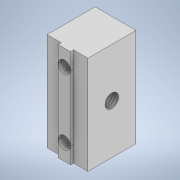
# Autodesk Inventor part: elbow clamp
Saved by Autodesk Inventor 2021 (Build 250183000, 183)
## iProperties
Created: 2022-09-09
Part Number: elbow clamp
Material: Generic
Document SubType Name: Modeling
Designer: szucs
Density: 1 g/cm^3
Appearance: Default
Author: szucs
Autodesk Inventor part; units mm, degrees
ref_plane "YZ Plane" through (0, 0, 0) normal (1, 0, 0) x (0, 1, 0)
ref_plane "XZ Plane" through (0, 0, 0) normal (0, 1, 0) x (-1, 0, 0)
ref_plane "XY Plane" through (0, 0, 0) normal (0, 0, 1) x (1, 0, 0)
sketch "Sketch1" plane through (0, 0, 0) normal (0, 0, 1) x (1, 0, 0)
  line L0 (0, 33.6) -> (0, -33.6) projected
  line L1 (-14, 0) -> (14, 0) projected
  line L2 (-10, 24) -> (10, 24)
  line L3 (10, 24) -> (10, -24)
  line L4 (10, -24) -> (-10, -24)
  line L5 (-10, -24) -> (-10, 24)
  point P0 (0, 0)
  dimension "d0" = 20
  dimension "d1" = 48
  constraints: 8 end point, 2 parallel, 1 horizontal, 1 perpendicular, 2 other
  measures "d0" distance of L3.end L4.end
  measures "d1" distance of L2.end L3.end
extrude "Extrusion1" add sketch "Sketch1" along normal blind 25
sketch "Sketch2" plane through (0, 0, 25) normal (0, 0, 1) x (1, 0, 0)
  line L0 (-10, -24) -> (10, -24) projected
  line L1 (10, -24) -> (10, 24) projected
  line L2 (10, 24) -> (-10, 24) projected
  line L3 (-10, 24) -> (-10, -24) projected
  line L4 (0, 47.04) -> (0, -47.04) projected
  line L5 (3, 33.6) -> (3, -33.6)
  line L6 (-3, 33.6) -> (-3, -33.6)
  point P0 (0, 0)
  point P1 (3, 24)
  point P2 (3, -24)
  point P3 (-3, -24)
  point P4 (-3, 24)
  dimension "d4" = 3
  dimension "d5" = 3
  constraints: 4 end point, 2 parallel
  measures "d4" distance between parallel lines of L4 L6
  measures "d5" distance between parallel lines of L4 L5
extrude "Extrusion2" cut sketch "Sketch2" against normal blind 1.5 contours L3 L2 L6 L0 | L5 L2 L1 L0
sketch "Sketch3" plane through (10, -24, 0) normal (1, 0, 0) x (0, 0, -1)
  line L0 (-30, 24) -> (5, 24) projected
  line L1 (-23.5, 48) -> (-23.5, 0) projected
  line L2 (0, 0) -> (-23.5, 0) projected
  line L3 (0, 0) -> (0, 48) projected
  line L4 (0, 48) -> (-23.5, 48) projected
  line L5 (-25, 0) -> (-25, 48) projected
  line L6 (-23.5, 0) -> (-25, 0) projected
  line L7 (-23.5, 0) -> (-23.5, 48) projected
  line L8 (-25, 48) -> (-23.5, 48) projected
  line L9 (0, 0) -> (-23.5, 0) projected
  line L10 (-11.75, 0) -> (-11.75, 48)
  line L11 (0, 48) -> (-23.5, 48) projected
  point P0 (0, 24)
  constraints: 2 end point, 2 midpoint
sketch "Sketch4" plane through (10, -24, 0) normal (1, 0, 0) x (0, 0, -1)
  point P0 (0, 24)
  point P1 (-11.8566, 24.141)
hole "Hole1" at (10, 0.141, 11.8566) direction (-1, 0, 0) diameter 6.647 end through all thread size "M8x1.25" class "6H" standard "ISO Metric profile"
sketch "Sketch5" plane through (0, 0, 25) normal (0, 0, 1) x (1, 0, 0)
  line L0 (3, -24) -> (3, 24) projected
  line L1 (3, 24) -> (-3, 24) projected
  line L2 (-3, 24) -> (-3, -24) projected
  line L3 (-3, -24) -> (3, -24) projected
  circle A0 centre (0, 16) radius 3
  circle A1 centre (0, -16) radius 3
  line L4 (0, 33.6) -> (0, -33.6) projected
  point P0 (0, 0)
  dimension "d15" = 6
  dimension "d16" = 6
  dimension "d17" = 8
  dimension "d18" = 8
  constraints: 2 centre point
  measures "d15" diameter of A0
  measures "d16" diameter of A1
  measures "d17" distance from line of L1 A0.centre
  measures "d18" distance from line of L3 A1.centre
extrude "Extrusion3" cut sketch "Sketch5" against normal through all contours A1 L4 | A0 L4 | L4 A1 | L4 A0
body "Solid1"
